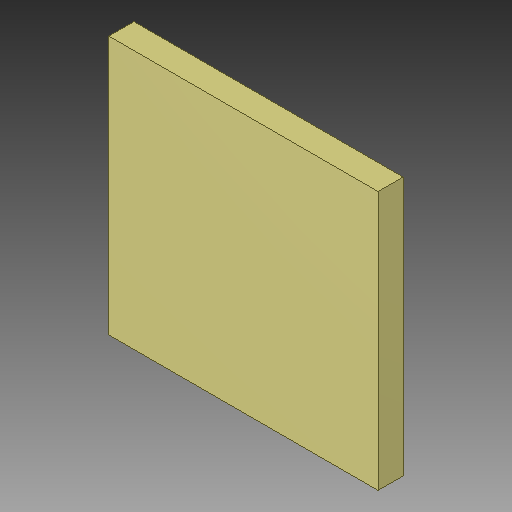
# Autodesk Inventor part: ATMEGA328PB-AUR
Saved by Autodesk Inventor 2017 (Build 210142000, 142)
## iProperties
Created: 2019-06-13
Part Number: ATMEGA328PB-AUR
Material: Generic
Document SubType Name: Modeling
Designer: Marc
Density: 1 g/cm^3
Appearance: QFP80P900X900X120-32N, ATMEGA328PB-AUR
Author: Marc
Autodesk Inventor part; units mm, degrees
ref_plane "YZ Plane" through (0, 0, 0) normal (1, 0, 0) x (0, 1, 0)
ref_plane "XZ Plane" through (0, 0, 0) normal (0, 1, 0) x (-1, 0, 0)
ref_plane "XY Plane" through (0, 0, 0) normal (0, 0, 1) x (1, 0, 0)
sketch "QFP80P900X900X120-32N, ATMEGA328PB-AUR_46" plane through (0, 0, 0) normal (0, 0, 1) x (1, 0, 0)
  line L0 (-5.573, 5.16) -> (5.16, 5.16)
  line L1 (5.16, 5.16) -> (5.16, -5.16)
  line L2 (5.16, -5.16) -> (-5.573, -5.16)
  line L3 (-5.573, -5.16) -> (-5.573, 5.16)
  constraints: 8 end point
extrude "Extrusion1" add sketch "QFP80P900X900X120-32N, ATMEGA328PB-AUR_46" along normal blind 1
body "Solid1"
